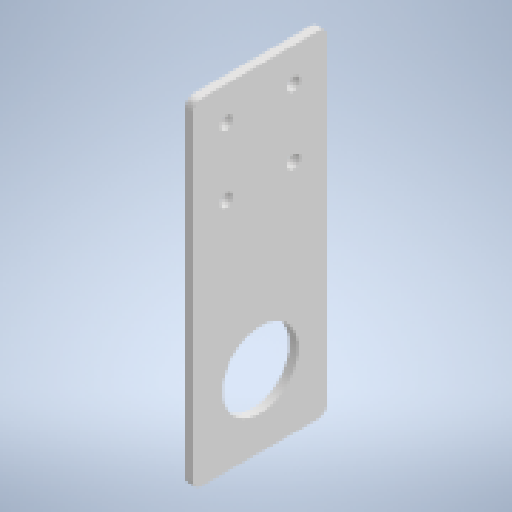
# Autodesk Inventor part: Drop for pivot intake
Saved by Autodesk Inventor 2023 (Build 270158000, 158)
## iProperties
Created: 2023-03-19
Part Number: Drop for pivot intake
Material: Generic
Document SubType Name: Modeling
Designer: Gabriel - T3 CAD
Density: 1 g/cm^3
Appearance: Default
Author: Gabriel - T3 CAD
Autodesk Inventor part; units mm, degrees
ref_plane "YZ Plane" through (0, 0, 0) normal (1, 0, 0) x (0, 1, 0)
ref_plane "XZ Plane" through (0, 0, 0) normal (0, 1, 0) x (-1, 0, 0)
ref_plane "XY Plane" through (0, 0, 0) normal (0, 0, 1) x (1, 0, 0)
sketch "Sketch1" plane through (0, 0, 0) normal (1, 0, 0) x (0, 1, 0)
  line L0 (-3.175, 0) -> (-123.825, 0)
  line L1 (-127, 3.175) -> (-127, 47.625)
  line L2 (-123.825, 50.8) -> (-3.175, 50.8)
  line L3 (0, 47.625) -> (0, 3.175)
  circle A0 centre (-100.0125, 25.4) radius 14.2875
  arc A1 (0, 47.625) -> (-3.175, 50.8) centre (-3.175, 47.625) ccw
  arc A2 (-3.175, 0) -> (0, 3.175) centre (-3.175, 3.175) ccw
  arc A3 (-127, 3.175) -> (-123.825, 0) centre (-123.825, 3.175) ccw
  arc A4 (-123.825, 50.8) -> (-127, 47.625) centre (-123.825, 47.625) ccw
  circle A5 centre (-12.7, 38.1) radius 2.3813
  circle A6 centre (-38.1, 38.1) radius 2.3813
  circle A7 centre (-63.5, 38.1) radius 2.3813
  circle A8 centre (-12.7, 12.7) radius 2.3813
  circle A9 centre (-38.1, 12.7) radius 2.3813
  circle A10 centre (-63.5, 12.7) radius 2.3813
  point P0 (0, 0)
  point P1 (-127, 50.8)
  point P2 (-127, 0)
  point P3 (0, 50.8)
  dimension "d0" = 127
  dimension "d1" = 50.8
  dimension "d4" = 26.9875
  dimension "d5" = 28.575
  dimension "d6" = 3.175
  dimension "d9" = 25.4
  dimension "d18" = 12.7
  dimension "d19" = 4.7625
  dimension "d20" = 12.7
  dimension "d23" = 25.4
  dimension "d26" = 25.4
  constraints: 11 centre point, 8 end point, 8 point on circle, 8 point on line, 8 tangent, 3 equal radius, 2 horizontal, 2 parallel, 1 perpendicular, 1 vertical, 10 other
  measures "d0" distance of point (-127, 50.8) point (0, 50.8)
  measures "d1" distance of point (-127, 0) point (-127, 50.8)
  measures "d4" distance from line of L1 A0.centre
  measures "d5" diameter of A0
  measures "d6" radius of A1
  measures "d9" distance from line of L0 A0.centre
  measures "d18" distance from line of L2 A5.centre
  measures "d19" diameter of A5
  measures "d20" distance from line of L3 A5.centre
  measures "d23" distance of A5.centre A6.centre
  measures "d26" distance of A5.centre A8.centre
extrude "Extrusion1" add sketch "Sketch1" along normal blind 3.175
equation "\"d9\" = 0.5 * d1"
equation "\"d18\" = -0.5 * d15 + 0.5 * d1"
equation "\"d15\" = 25.4"
body "Solid1"
